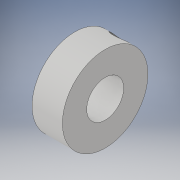
# Autodesk Inventor part: 6mm rod topper
Saved by Autodesk Inventor 2019 (Build 230136000, 136)
## iProperties
Created: 2019-06-10
Part Number: 6mm rod topper
Material: Generic
Document SubType Name: Modeling
Designer: Matthew XPS
Density: 1 g/cm^3
Appearance: Default
Author: Matthew XPS
Autodesk Inventor part; units mm, degrees
ref_plane "YZ Plane" through (0, 0, 0) normal (1, 0, 0) x (0, 1, 0)
ref_plane "XZ Plane" through (0, 0, 0) normal (0, 1, 0) x (-1, 0, 0)
ref_plane "XY Plane" through (0, 0, 0) normal (0, 0, 1) x (1, 0, 0)
sketch "Sketch1" plane through (0, 0, 0) normal (1, 0, 0) x (0, 1, 0)
  circle A0 centre (0, 0) radius 3.05
  circle A1 centre (0, 0) radius 7.05
  dimension "d0" = 6.1
  dimension "d1" = 4
  constraints: 2 centre point, 1 coincident
  measures "d0" diameter of A0
  measures "d1" radial gap between concentric circles of A0 A1
extrude "Extrusion1" add sketch "Sketch1" along normal blind 5
sketch "Sketch2" plane through (5, 0, 0) normal (1, 0, 0) x (0, 0, -1)
  line L0 (0, 0) -> (4.9851, 4.9851)
  circle A0 centre (0, 0) radius 7.05 projected
  line L1 (0, 0) -> (7.05, 0) construction
  dimension "d4" = 45
  constraints: 4 end point, 1 equal length, 1 horizontal, 2 other
  measures "d4" angle of L1 L0
ref_plane "Work Plane1" through (5, 4.9851, -4.9851) normal (0, 0.7071068, -0.7071068) x (-1, 0, 0)
sketch "Sketch3" plane through (5, 4.9851, -4.9851) normal (0, 0.7071068, -0.7071068) x (-1, 0, 0)
  line L0 (5, 0) -> (0, 0)
  line L1 (0, 7.05) -> (0, -7.05) projected
  line L2 (5, 0) -> (10, 0) construction
  circle A0 centre (2.5, 0) radius 1.5
  dimension "d5" = 5
  dimension "d6" = 180
  dimension "d7" = 3
  constraints: 4 end point, 1 centre point, 1 collinear, 1 horizontal, 1 midpoint, 1 perpendicular
  measures "d5" distance of L0.start L0.end
  measures "d6" angle of L0 L2
  measures "d7" diameter of A0
extrude "Extrusion2" cut sketch "Sketch3" against normal blind 5
thread "Thread1" size "M3x0.5" class "6H" standard "ANSI Metric M Profile" full length
body "Solid1"
